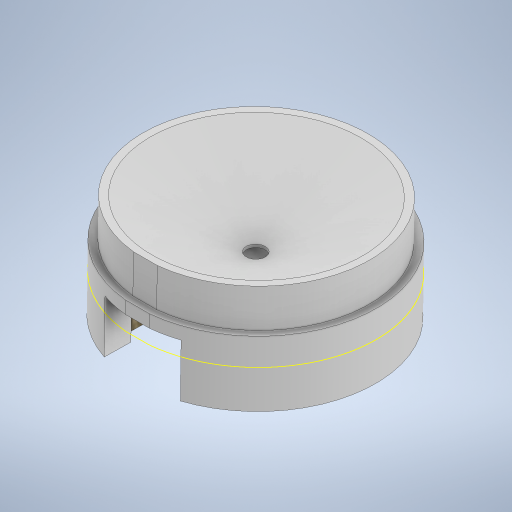
# Autodesk Inventor part: PiezoMount
Saved by Autodesk Inventor 2023 (Build 270158000, 158)
## iProperties
Created: 2023-02-27
Part Number: PiezoMount
Material: Generic
Document SubType Name: Modeling
Designer: maste
Density: 1 g/cm^3
Appearance: Default
Author: maste
Autodesk Inventor part; units mm, degrees
ref_plane "YZ Plane" through (0, 0, 0) normal (1, 0, 0) x (0, 1, 0)
ref_plane "XY Plane" through (0, 0, 0) normal (0, 0, 1) x (1, 0, 0)
sketch "Sketch1" plane through (0, 0, 0) normal (0, 0, 1) x (1, 0, 0)
  circle A0 centre (0, 0) radius 25
  dimension "d2" = 50
  constraints: 1 centre point, 1 coincident
  measures "d2" diameter of A0
extrude "piezo surface" add sketch "Sketch1" along normal blind 8
sketch "Sketch4" plane through (0, 0, 0) normal (0, 0, -1) x (-1, 0, 0)
  circle A0 centre (0, 0) radius 25 projected
extrude "Depth extension to surface" add sketch "Sketch4" along normal blind 3.62
sketch "Sketch2" plane through (0, 0, 8) normal (0, 0, 1) x (1, 0, 0)
  circle A0 centre (0, 0) radius 17.95
  circle A1 centre (0, 0) radius 18.75
  line L0 (0, 0) -> (18.75, 0)
  arc A2 (18.75, 0) -> (16.238, 9.375) centre (0, 0) ccw
  line L1 (0, 0) -> (16.238, 9.375) construction
  line L2 (0, 0) -> (18.75, 0) construction
  line L3 (16.238, 9.375) -> (15.5452, 8.975)
  line L4 (0, 0) -> (0, 18.75)
  line L5 (0, 0) -> (0, -18.75)
  line L6 (0, 0) -> (-18.75, 0)
  line L7 (0, 0) -> (-16.238, -9.375)
  line L8 (0, 0) -> (-9.375, 16.238)
  line L9 (0, 0) -> (9.375, -16.238)
  point P0 (17.95, 0)
  point P1 (8.975, -15.5452)
  point P2 (0, -17.95)
  point P3 (-15.5452, -8.975)
  point P4 (-17.95, 0)
  point P5 (-8.975, 15.5452)
  point P6 (0, 17.95)
  dimension "d3" = 35.9
  dimension "d4" = 37.5
  dimension "d5" = 30
  constraints: 20 end point, 4 point on line, 3 coincident, 2 perpendicular, 2 point on circle, 1 centre point, 1 horizontal, 1 vertical, 12 other
  measures "d5" angle of L2 L1
sketch "Sketch3" plane through (0, 0, 8) normal (0, 0, 1) x (1, 0, 0)
  line L0 (0, 0) -> (8.975, -15.5452)
  arc A0 (17.95, 0) -> (15.5452, 8.975) centre (0, 0) ccw projected
  line L1 (0, 0) -> (17.95, 0)
  arc A1 (0, -17.95) -> (8.975, -15.5452) centre (0, 0) ccw projected
  line L2 (8.975, -15.5452) -> (17.95, 0)
  line L3 (13.4625, -7.7726) -> (0, 0)
  line L4 (13.4625, -7.7726) -> (4.8022, -2.7726)
  line L5 (13.4625, -7.7726) -> (4.8022, -2.7726)
  line L6 (13.4625, -7.7726) -> (4.8022, -2.7726)
  line L7 (4.8022, -2.7726) -> (6.0522, -0.6075)
  line L8 (6.0522, -0.6075) -> (14.7125, -5.6075)
  line L9 (14.7125, -5.6075) -> (13.4625, -7.7726)
  line L10 (13.4625, -7.7726) -> (4.8022, -2.7726)
  line L11 (4.8022, -2.7726) -> (3.5522, -4.9376)
  line L12 (3.5522, -4.9376) -> (12.2125, -9.9376)
  line L13 (12.2125, -9.9376) -> (13.4625, -7.7726)
  line L14 (12.2125, -9.9376) -> (14.7125, -5.6075)
  line L15 (14.7125, -5.6075) -> (16.4446, -6.6075)
  line L16 (16.4446, -6.6075) -> (13.9446, -10.9376)
  line L17 (13.9446, -10.9376) -> (12.2125, -9.9376)
  line L18 (-4.802, 2.7724) -> (-3.552, 4.9375)
  line L19 (-3.552, 4.9375) -> (-13.9443, 10.9375)
  line L20 (-4.802, 2.7724) -> (-6.052, 0.6074)
  line L21 (-6.052, 0.6074) -> (-16.4443, 6.6074)
  line L22 (-16.4443, 6.6074) -> (-23.8055, 10.8574)
  line L23 (-23.8055, 10.8574) -> (-21.3055, 15.1875)
  line L24 (-21.3055, 15.1875) -> (-13.9443, 10.9375)
  line L25 (-5.5448, 2.5) -> (-17.5448, 2.5)
  line L26 (-5.5448, 0) -> (-5.5448, 2.5)
  line L27 (-5.5448, 0) -> (-5.5448, -2.5)
  line L28 (-5.5448, -2.5) -> (-17.5448, -2.5)
  line L29 (-17.5448, -2.5) -> (-26.0448, -2.5)
  line L30 (-26.0448, -2.5) -> (-26.0448, 2.5)
  line L31 (-26.0448, 2.5) -> (-17.5448, 2.5)
  point P0 (14.7125, -5.6075)
  point P1 (12.2125, -9.9376)
  point P2 (12.2125, -9.9376)
  dimension "d37" = 10
  dimension "d38" = 2.5
  dimension "d39" = 2.5
  dimension "d40" = 2
  dimension "d49" = 10
  dimension "d69" = 30
  dimension "d71" = 20.5
  dimension "d72" = 5
  constraints: 64 end point, 7 parallel, 4 collinear, 3 perpendicular, 1 midpoint, 1 point on line, 15 other
  measures "d37" distance of L3.start L4.end
  measures "d38" distance of L4.end L7.end
  measures "d39" distance of L11.end L4.end
  measures "d40" distance of L8.end L15.end
  measures "d49" distance between parallel lines of L11 L13
  measures "d71" distance between parallel lines of L30 L27
  measures "d72" distance between parallel lines of L25 L28
extrude "Microphone Wire Hole" cut sketch "Sketch3" against normal blind 14 contours L26 L27 L28 L29 L30 L31 L25 L21 L20 | L20 L21 L25 L26
sketch "Sketch5" plane through (0, 0, -3.62) normal (0, 0, -1) x (-1, 0, 0)
  line L0 (16, -16) -> (-16, -16)
  line L1 (-16, -16) -> (-16, 16)
  line L2 (-16, 16) -> (16, 16)
  line L3 (16, 16) -> (16, -16)
  line L4 (16, -16) -> (-16, 16) construction
  line L5 (-16, -16) -> (16, 16) construction
  circle A0 centre (0, 0) radius 20
  point P0 (-12, -16)
  point P1 (12, -16)
  point P2 (-16, 12)
  point P3 (-16, -12)
  point P4 (16, 12)
  point P5 (16, -12)
  point P6 (12, 16)
  point P7 (-12, 16)
  dimension "d18" = 32
  dimension "d19" = 32
  dimension "d54" = 40
  constraints: 12 end point, 2 midpoint, 2 parallel, 1 centre point, 1 coincident, 1 horizontal, 1 perpendicular
  measures "d18" distance of L0.start L0.end
  measures "d19" distance of L0.end L1.end
  measures "d54" diameter of A0
extrude "Circuit chamber" cut sketch "Sketch5" against normal blind 3
sketch "Sketch6" plane through (-16, -16, -3.62) normal (1, 0, 0) x (0, 0, -1)
  line L0 (0, 4) -> (0, 0) projected
  line L1 (0, 32) -> (-3, 32) projected
  line L2 (-3, 32) -> (-3, 28) projected
  line L3 (0, 0) -> (-3, 0) projected
  line L4 (-3, 4) -> (-3, 0) projected
  line L5 (0, 32) -> (0, 28) projected
  line L6 (0, 4) -> (-3, 4) projected
  line L7 (0, 18.5) -> (0, 13.5) projected
  line L8 (-11.62, 13.5) -> (-11.62, 18.5) projected
  line L9 (-3, 32) -> (-3, 28) projected
  line L10 (-3, 32) -> (-3, 32) projected
  line L11 (-3, 28) -> (-3, 32) projected
  line L12 (-3, 4) -> (-3, 28) projected
  line L13 (-3, 0) -> (-3, 4) projected
  line L14 (-3, 0) -> (-3, 0) projected
  line L15 (-3, 4) -> (-3, 0) projected
  line L16 (-3, 13.5) -> (-3, 4) projected
  line L17 (0, 18.5) -> (0, 13.5) projected
  line L18 (0, 13.5) -> (0, 4) projected
  line L19 (0, 4) -> (0, 0) projected
  line L20 (0, 0) -> (0, 0) projected
  line L21 (0, 0) -> (0, 4) projected
  line L22 (0, 4) -> (0, 28) projected
  line L23 (0, 28) -> (0, 32) projected
  line L24 (0, 32) -> (0, 32) projected
  line L25 (0, 32) -> (0, 28) projected
  line L26 (-11.62, 16) -> (0, 16)
  line L27 (0, 16) -> (-3, 16)
  line L28 (-3, 16) -> (-3, 24)
  line L29 (-3, 24) -> (0, 24)
  line L30 (0, 24) -> (0, 16)
  line L31 (0, 16) -> (-3, 16)
  line L32 (-3, 16) -> (-3, 8)
  line L33 (-3, 8) -> (0, 8)
  line L34 (0, 8) -> (0, 16)
  line L35 (0, 28) -> (0, 18.5) projected
  line L36 (-3, 18.5) -> (-3, 13.5) projected
  line L37 (-3, 28) -> (-3, 18.5) projected
  line L38 (0, 28) -> (-3, 28) projected
  line L39 (0, 18.5) -> (-11.62, 18.5) projected
  line L40 (-11.62, 13.5) -> (0, 13.5) projected
  point P0 (0, -9)
  point P1 (0, 41)
  point P2 (-11, 41)
  point P3 (-11, -9)
  point P4 (0, -9)
  point P5 (0, 41)
  point P6 (-3, 4)
  point P7 (-3, 8)
  point P8 (0, 8)
  point P9 (-3, 16)
  point P10 (-3, 13.5)
  point P11 (0, 13.5)
  point P12 (0, 18.5)
  dimension "d65" = 8
  dimension "d66" = 8
  constraints: 18 end point, 4 parallel, 2 horizontal, 2 midpoint, 2 perpendicular, 2 point on line
  measures "d65" distance of L27.end L28.end
  measures "d66" distance of L32.end L31.end
extrude "port vent" cut sketch "Sketch6" against normal blind 30 contours L33 L12 L40 L18 | L39 L12 L29 L22
sketch "Sketch7" plane through (0, 0, -3.62) normal (0, 0, -1) x (-1, 0, 0)
  line L0 (0, 0) -> (0, -17.5)
  line L1 (0, 0) -> (0, 17.5)
  dimension "d25" = 17.5
  dimension "d26" = 17.5
  constraints: 4 end point, 2 coincident, 2 vertical
  measures "d25" distance of L0.start L0.end
  measures "d26" distance of L0.start L1.end
hole "screw holes" at (0, 17.5, -3.62) at (0, -17.5, -3.62) direction (0, 0, 1) diameter 3.7 depth 4 tip angle 118
sketch "Sketch8" plane through (0, 0, -3.62) normal (0, 0, -1) x (-1, 0, 0)
  circle A0 centre (0, 0) radius 22.75
  line L0 (21.4137, 11) -> (22.4499, 11) projected
  line L1 (22.4499, 11) -> (19.9139, 11)
  arc A1 (23.6854, 8) -> (23.6854, -8) centre (0, 0) ccw projected
  line L2 (24.6779, -4) -> (22.3956, -4)
  arc A2 (24.8747, 2.5) -> (24.8747, -2.5) centre (0, 0) ccw projected
  arc A3 (-16, 12) -> (-16, -12) centre (0, 0) ccw projected
  arc A4 (-12, -16) -> (12, -16) centre (0, 0) ccw projected
  point P0 (12.5, 7.5)
  point P1 (15.0629, 9)
  point P2 (19.2094, 16)
  point P3 (19.2094, -16)
  point P4 (19.9139, 11)
  point P5 (16.7033, 11)
  point P6 (24.6779, 4)
  point P7 (21.9317, -12)
  dimension "d34" = 45.5
  constraints: 4 end point, 2 point on circle, 1 centre point, 1 coincident, 1 horizontal, 1 parallel, 1 other
  measures "d34" diameter of A0
sketch "Sketch10" plane through (0, 0, -3.62) normal (0, 0, -1) x (-1, 0, 0)
  arc A0 (23.6854, 8) -> (23.6854, -8) centre (0, 0) ccw projected
  arc A1 (16, -12) -> (18.3303, -8) centre (0, 0) ccw projected
  line L0 (16, -16) -> (12, -16) projected
  arc A2 (-12, -16) -> (12, -16) centre (0, 0) ccw projected
  line L1 (-12, -16) -> (-16, -16) projected
  line L2 (-16, -16) -> (-16, -12) projected
  arc A3 (-16, 12) -> (-16, -12) centre (0, 0) ccw projected
  line L3 (-16, 12) -> (-16, 16) projected
  line L4 (-16, 16) -> (-12, 16) projected
  arc A4 (12, 16) -> (-12, 16) centre (0, 0) ccw projected
  line L5 (12, 16) -> (16, 16) projected
  line L6 (16, 16) -> (16, 12) projected
  line L7 (18.3303, 8) -> (23.6854, 8) projected
  line L8 (23.6854, -8) -> (18.3303, -8) projected
  line L9 (16, -12) -> (16, -16) projected
  arc A5 (18.3303, 8) -> (16, 12) centre (0, 0) ccw projected
extrude "Base Extension" add sketch "Sketch10" along normal blind 10
sketch "Sketch13" plane through (0, 0, 8) normal (0, 0, 1) x (0, 1, 0)
  circle A0 centre (0, 0) radius 25
  circle A1 centre (0, 0) radius 23.5
  dimension "d55" = 47
  dimension "d59" = 50
  constraints: 2 centre point, 2 coincident
  measures "d55" diameter of A1
  measures "d59" diameter of A0
extrude "Rim for flush with diaphragm lock" cut sketch "Sketch13" against normal blind 8
sketch "Sketch14" plane through (-16, 12.1244, -3) normal (1, 0, 0) x (0, 0, -1)
  line L0 (10.62, -4.1244) -> (10.62, -20.1244) projected
  line L1 (-3, 11.3756) -> (-11, 11.3756) projected
  line L2 (-11, 11.3756) -> (-11, -35.6244) projected
  line L3 (-3, -9.6244) -> (-3, -14.6244) projected
  line L4 (-2.38, -20.1244) -> (10.62, -20.1244) projected
  line L5 (10.62, -4.1244) -> (-2.38, -4.1244) projected
  line L6 (-3, -14.6244) -> (-2.38, -14.6244) projected
  line L7 (-2.38, -14.6244) -> (-2.38, -20.1244) projected
  line L8 (-2.38, -4.1244) -> (-2.38, -9.6244) projected
  line L9 (-2.38, -9.6244) -> (-3, -9.6244) projected
  point P0 (-3, -12.1244)
  point P1 (-4, -2.6061)
  point P2 (-4, 1.724)
  point P3 (-11, -35.6244)
  constraints: 1 other
sketch "Sketch16" plane through (0, 0, 8) normal (0, 0, 1) x (1, 0, 0)
  circle A0 centre (0, 0) radius 18
  arc A1 (-23.3666, -2.5) -> (-23.3666, 2.5) centre (0, 0) ccw projected
  line L0 (-23.3666, 2.5) -> (-5.5448, 2.5) projected
  line L1 (-5.5448, 2.5) -> (-5.5448, -2.5) projected
  line L2 (-5.5448, -2.5) -> (-23.3666, -2.5) projected
  point P0 (-17.8255, -2.5)
  point P1 (-17.8255, 2.5)
  dimension "d73" = 36
  constraints: 1 centre point, 1 coincident
  measures "d73" diameter of A0
extrude "Extrusion11" add sketch "Sketch16" along normal blind 1 contours A0 L2 L1 L0 picked at (2.3035, 0)
sketch "Sketch17" plane through (0, 0, -13.62) normal (0, 0, -1) x (-1, 0, 0)
  arc A0 (12, 16) -> (-12, 16) centre (0, 0) ccw projected
  line L0 (12, 16) -> (-12, 16)
  line L1 (-12, 20.5) -> (12, 20.5)
  line L2 (12, 20.5) -> (12, 11.5)
  line L3 (12, 11.5) -> (-12, 11.5)
  line L4 (-12, 11.5) -> (-12, 20.5)
  line L5 (-12, 20.5) -> (12, 11.5) construction
  line L6 (12, 20.5) -> (-12, 11.5) construction
  arc A1 (-16, 12) -> (-16, -12) centre (0, 0) ccw projected
  line L7 (0, 0) -> (-20, 0)
  line L8 (-12, -20.5) -> (12, -20.5)
  line L9 (12, -20.5) -> (12, -11.5)
  line L10 (12, -11.5) -> (-12, -11.5)
  line L11 (-12, -11.5) -> (-12, -20.5)
  point P0 (0, 16)
  dimension "d76" = 9
  constraints: 24 end point, 4 symmetric about line, 3 midpoint, 2 parallel, 1 horizontal, 1 perpendicular, 1 point on circle
  measures "d76" distance of L1.end L2.end
extrude "Extrusion12" add sketch "Sketch17" against normal blind 4
fillet "Fillet1" radius 5 4 edges at (-12, -11.5, -11.62) (12, -11.5, -11.62) (12, 11.5, -11.62) (-12, 11.5, -11.62)
sketch "Sketch18" plane through (0, 0, -13.62) normal (0, 0, -1) x (-1, 0, 0)
  circle A0 centre (0, -17.5) radius 1.85 projected
  circle A1 centre (0, 17.5) radius 1.85 projected
  arc A2 (23.6854, 8) -> (23.6854, -8) centre (0, 0) ccw projected
  dimension "d87" = 17.5
  dimension "d88" = 17.5
  dimension "d92" = 3.7
  measures "d87" distance of A2.centre A1.centre
  measures "d88" distance of point (0, 0) A0.centre
  measures "d92" diameter of A0
extrude "Extrusion13" cut sketch "Sketch18" against normal blind 4
sketch "Sketch19" plane through (0, 0, -9.62) normal (0, 0, 1) x (1, 0, 0)
  circle A0 centre (0, 17.5) radius 1.85 projected
  arc A1 (-12, 16) -> (-7.0251, 11.5) centre (-7.0251, 16.5) ccw projected
  line L0 (-7.0251, 11.5) -> (7.0251, 11.5) projected
  arc A2 (7.0251, 11.5) -> (12, 16) centre (7.0251, 16.5) ccw projected
  arc A3 (12, 16) -> (-12, 16) centre (0, 0) ccw projected
  line L1 (-1.2512, 20.6061) -> (2.0643, 20.1366)
  circle A4 centre (0, -17.5) radius 1.85 projected
  arc A5 (12, -16) -> (7.0251, -11.5) centre (7.0251, -16.5) ccw projected
  line L2 (7.0251, -11.5) -> (-7.0251, -11.5) projected
  arc A6 (-7.0251, -11.5) -> (-12, -16) centre (-7.0251, -16.5) ccw projected
  arc A7 (-12, -16) -> (12, -16) centre (0, 0) ccw projected
  circle A8 centre (0, -17.5) radius 1.85 projected
  line L3 (3.5218, -17.5) -> (1.7609, -20.55)
  line L4 (1.7609, -20.55) -> (-1.7609, -20.55)
  line L5 (-1.7609, -20.55) -> (-3.5218, -17.5)
  line L6 (-3.5218, -17.5) -> (-1.7609, -14.45)
  line L7 (-1.7609, -14.45) -> (1.7609, -14.45)
  line L8 (1.7609, -14.45) -> (3.5218, -17.5)
  line L9 (1.7609, 20.55) -> (3.5218, 17.5)
  line L10 (3.5218, 17.5) -> (1.7609, 14.45)
  line L11 (1.7609, 14.45) -> (-1.7609, 14.45)
  line L12 (-1.7609, 14.45) -> (-3.5218, 17.5)
  line L13 (-3.5218, 17.5) -> (-1.7609, 20.55)
  line L14 (-1.7609, 20.55) -> (1.7609, 20.55)
  point P0 (-2.1451, -19.8846)
  point P1 (2.1451, -19.8846)
  dimension "d83" = 6.1
  dimension "d86" = 6.1
  dimension "d209" = 0
  constraints: 26 end point, 3 coincident, 28 other
  measures "d83" distance between parallel lines of L6 L3
  measures "d86" distance between parallel lines of L12 L9
  measures "d209" angle of L2 L7
extrude "Extrusion14" cut sketch "Sketch19" against normal blind 1 contours A0 | L13 L14 L1 L9 A3 | A3 L9 L10 L11 L12 L13 | L1 L14 L9 | L3 L4 L5 A7 | A7 L5 L6 L7 L8 L3
sketch "Sketch20" plane through (0, 0, -0.62) normal (0, 0, -1) x (-1, 0, 0)
  circle A0 centre (0, 17.5) radius 1.85 projected
  line L0 (-1.7609, 14.45) -> (1.7609, 14.45) projected
  line L1 (-3.5218, 17.5) -> (-1.7609, 14.45) projected
  line L2 (-1.7609, 20.55) -> (-3.5218, 17.5) projected
  line L3 (1.7609, 20.55) -> (-1.7609, 20.55) projected
  line L4 (3.5218, 17.5) -> (1.7609, 20.55) projected
  line L5 (1.7609, 14.45) -> (3.5218, 17.5) projected
  line L6 (1.7609, -14.45) -> (-1.7609, -14.45) projected
  line L7 (3.5218, -17.5) -> (1.7609, -14.45) projected
  line L8 (1.7609, -20.55) -> (3.5218, -17.5) projected
  line L9 (-3.5218, -17.5) -> (-1.7609, -20.55) projected
  line L10 (-1.7609, -14.45) -> (-3.5218, -17.5) projected
  circle A1 centre (0, -17.5) radius 1.85 projected
  line L11 (-1.7609, -20.55) -> (1.7609, -20.55) projected
  point P0 (0, 0)
  dimension "d91" = 6.1
  measures "d91" distance between parallel lines of L9 L7
extrude "Extrusion15" cut sketch "Sketch20" along normal blind 11 contours L1 L2 L3 L4 L5 L0 | L7 L8 L11 L9 L10 L6 | A1
ref_plane "Work Plane3" through (0, 23.5, 0) normal (0, 1, 0) x (-1, 0, 0)
sketch "Sketch28" plane through (0, 0, -13.62) normal (0, 0, -1) x (-1, 0, 0)
  point P0 (0, 0)
sketch "Sketch27" plane through (0, 0, -0.62) normal (0, 0, -1) x (-1, 0, 0)
  circle A0 centre (0, 17.5) radius 1.85 projected
  circle A1 centre (0, -17.5) radius 1.85 projected
  arc A2 (7.0251, 11.5) -> (12, 16) centre (7.0251, 16.5) ccw projected
  line L0 (12, 16) -> (16, 16) projected
  line L1 (16, 16) -> (16, 12) projected
  arc A3 (18.3303, 8) -> (16, 12) centre (0, 0) ccw projected
  line L2 (18.3303, 8) -> (23.6854, 8) projected
  arc A4 (23.6854, 8) -> (23.6854, -8) centre (0, 0) ccw projected
  line L3 (23.6854, -8) -> (18.3303, -8) projected
  arc A5 (16, -12) -> (18.3303, -8) centre (0, 0) ccw projected
  line L4 (16, -12) -> (16, -16) projected
  line L5 (16, -16) -> (12, -16) projected
  arc A6 (12, -16) -> (7.0251, -11.5) centre (7.0251, -16.5) ccw projected
  line L6 (7.0251, -11.5) -> (-7.0251, -11.5) projected
  arc A7 (-7.0251, -11.5) -> (-12, -16) centre (-7.0251, -16.5) ccw projected
  line L7 (-12, -16) -> (-16, -16) projected
  line L8 (-16, -16) -> (-16, -12) projected
  arc A8 (-16, 12) -> (-16, -12) centre (0, 0) ccw projected
  line L9 (-16, 12) -> (-16, 16) projected
  line L10 (-16, 16) -> (-12, 16) projected
  arc A9 (-12, 16) -> (-7.0251, 11.5) centre (-7.0251, 16.5) ccw projected
  line L11 (-7.0251, 11.5) -> (7.0251, 11.5) projected
  line L12 (18.3303, 8) -> (-3.4197, 8)
  line L13 (-3.4197, 8) -> (-3.4197, -8)
  line L14 (-3.4197, -8) -> (18.3303, -8)
  line L15 (18.3303, -8) -> (18.3303, 8)
  line L16 (-3.4197, 0) -> (16.0803, 0)
  line L17 (16.0803, 0) -> (16.0803, 10)
  line L18 (16.0803, 10) -> (-3.4197, 10)
  line L19 (-3.4197, 10) -> (-3.4197, 0)
  line L20 (-3.4197, 0) -> (16.0803, 0)
  line L21 (16.0803, 0) -> (16.0803, -10)
  line L22 (16.0803, -10) -> (-3.4197, -10)
  line L23 (-3.4197, -10) -> (-3.4197, 0)
  line L24 (20.3303, -11.5) -> (20.3303, 11.5)
  line L25 (20.3303, 11.5) -> (-7.6697, 11.5)
  line L26 (-7.6697, 11.5) -> (-7.6697, -11.5)
  line L27 (-7.6697, -11.5) -> (20.3303, -11.5)
  line L28 (20.3303, -11.5) -> (-7.6697, 11.5) construction
  line L29 (20.3303, 11.5) -> (-7.6697, -11.5) construction
  point P0 (6.3303, 0)
  point P1 (-7.0251, -11.5)
  point P2 (16.3631, -11.5)
  point P3 (17.3205, -10)
  point P4 (17.3205, 10)
  point P5 (16.3631, 11.5)
  point P6 (16.0803, 8)
  point P7 (16.0803, -8)
  point P8 (20.3303, 8)
  point P9 (20.3303, -8)
  dimension "d132" = 21.75
  dimension "d133" = 16
  dimension "d134" = 10
  dimension "d135" = 10
  dimension "d136" = 28
  constraints: 36 end point, 8 parallel, 4 midpoint, 4 perpendicular, 3 horizontal, 1 point on line, 1 vertical
  measures "d132" distance of L14.end L13.end
  measures "d133" distance of L14.end L2.start
  measures "d134" distance of L17.end L16.end
  measures "d135" distance of L20.end L21.end
  measures "d136" distance of L25.end L24.end
extrude "Extrusion20" add sketch "Sketch27" along normal blind 5 contours L25 A3 L12 L17 L18 L19 L13 L23 L22 L21 L14 A5 L27 L6 L26 L11 | A2 L0 L1 A3 L25 | L25 L24 L2 A3 | L3 L24 L27 A5
sketch "Sketch30" plane through (0, 0, -0.62) normal (0, 0, -1) x (-1, 0, 0)
  line L0 (16.0803, 10) -> (-3.4197, 10) projected
  line L1 (-3.4197, 10) -> (-3.4197, -10) projected
  line L2 (-3.4197, -10) -> (16.0803, -10) projected
  arc A0 (12, 16) -> (2.1451, 19.8846) centre (0, 0) ccw projected
  line L3 (16.0803, -8) -> (23.6854, -8) projected
  line L4 (5.5448, -2.5) -> (24.8747, -2.5) projected
  line L5 (5.5448, 2.5) -> (5.5448, -2.5) projected
  line L6 (24.8747, 2.5) -> (5.5448, 2.5) projected
  line L7 (23.6854, 8) -> (16.0803, 8) projected
  arc A1 (-12, -16) -> (-2.1451, -19.8846) centre (0, 0) ccw projected
  arc A2 (23.6854, -8) -> (24.8747, -2.5) centre (0, 0) ccw projected
  arc A3 (24.8747, 2.5) -> (23.6854, 8) centre (0, 0) ccw projected
  line L8 (16.3631, -11.5) -> (-7.6697, -11.5) projected
  line L9 (-7.6697, -11.5) -> (-7.6697, 11.5) projected
  line L10 (-7.6697, 11.5) -> (7.0251, 11.5) projected
  arc A4 (7.0251, 11.5) -> (12, 16) centre (7.0251, 16.5) ccw projected
  line L11 (2.1451, 19.8846) -> (1.7609, 20.55) projected
  line L12 (1.7609, 20.55) -> (-1.7609, 20.55) projected
  line L13 (-1.7609, 20.55) -> (-2.1451, 19.8846) projected
  arc A5 (2.1451, -19.8846) -> (12, -16) centre (0, 0) ccw projected
  line L14 (-16, 16) -> (-12, 16) projected
  line L15 (-16, 12) -> (-16, 16) projected
  line L16 (-16, -16) -> (-16, -12) projected
  line L17 (-12, -16) -> (-16, -16) projected
  arc A6 (-2.1451, 19.8846) -> (-12, 16) centre (0, 0) ccw projected
  line L18 (-2.1451, -19.8846) -> (-1.7609, -20.55) projected
  line L19 (-1.7609, -20.55) -> (1.7609, -20.55) projected
  line L20 (1.7609, -20.55) -> (2.1451, -19.8846) projected
  arc A7 (-16, 12) -> (-16, -12) centre (0, 0) ccw projected
  line L21 (16, -16) -> (12, -16) projected
  line L22 (16, -12) -> (16, -16) projected
  arc A8 (16, -12) -> (16.3631, -11.5) centre (0, 0) ccw projected
  line L23 (16.0803, 8) -> (16.0803, 10) projected
  line L24 (16.0803, -10) -> (16.0803, -8) projected
extrude "Extrusion21" add sketch "Sketch30" along normal blind 2 contours L23 L7 A3 L6 L5 L4 A2 L3 L24 L2 L1 L0
sketch "Sketch31" plane through (0, 0, 9) normal (0, 0, 1) x (1, 0, 0)
  circle A0 centre (0, 0) radius 2
  dimension "d153" = 4
  constraints: 1 centre point, 1 coincident
  measures "d153" diameter of A0
extrude "Extrusion22" cut sketch "Sketch31" against normal blind 15
chamfer "Chamfer10" distance 0.5 angle 45 2 edges at (0, 14.45, -9.62) (0, -14.45, -9.62)
chamfer "Chamfer11" distance 0.5 angle 45 8 edges at (-1.6166, -14.2, -9.62) (-2.6414, -15.975, -9.62) (1.6166, -14.2, -9.62) (2.6414, -15.975, -9.62) (-1.6166, 14.2, -9.62) (-2.6414, 15.975, -9.62) (1.6166, 14.2, -9.62) (2.6414, 15.975, -9.62)
sketch "Sketch49" plane through (0, 0, -5.62) normal (0, 0, -1) x (-1, 0, 0)
  line L0 (17.5701, -10.7544) -> (5.518, -10.7544)
  line L1 (5.518, -10.7544) -> (5.518, -16.7393)
  line L2 (5.518, -16.7393) -> (17.5701, -16.7393)
  line L3 (17.5701, -16.7393) -> (17.5701, -10.7544)
  point P0 (0, 0)
  constraints: 8 end point, 2 parallel, 1 horizontal, 1 perpendicular
extrude "Extrusion37" add sketch "Sketch49" against normal blind 2.97
sketch "Sketch50" plane through (0, 0, -9.62) normal (0, 0, 1) x (1, 0, 0)
  arc A0 (12, 16) -> (2.1451, 19.8846) centre (0, 0) ccw projected
  line L0 (2.1451, 19.8846) -> (4.6765, 15.5) projected
  line L1 (4.6765, 15.5) -> (3.7816, 13.95) projected
  line L2 (7.0251, 11.5) -> (-2.0496, 11.5) projected
  arc A1 (7.0251, 11.5) -> (12, 16) centre (7.0251, 16.5) ccw projected
  line L3 (-2.0496, -11.5) -> (7.0251, -11.5) projected
  line L4 (3.7816, -13.95) -> (4.6765, -15.5) projected
  line L5 (4.6765, -15.5) -> (2.1451, -19.8846) projected
  arc A2 (2.1451, -19.8846) -> (12, -16) centre (0, 0) ccw projected
  arc A3 (12, -16) -> (7.0251, -11.5) centre (7.0251, -16.5) ccw projected
  line L6 (7.6697, -11.5) -> (-5.518, -11.5) projected
  line L7 (7.6697, -2.275) -> (7.6697, -11.5) projected
  arc A4 (3.4197, -7.2323) -> (7.6697, -2.275) centre (0, 0) ccw projected
  line L8 (3.4197, -10) -> (3.4197, -7.2323) projected
  line L9 (-16.0803, -10) -> (3.4197, -10) projected
  line L10 (-16.0803, -8) -> (-16.0803, -10) projected
  line L11 (-23.6854, -8) -> (-16.0803, -8) projected
  arc A5 (-23.6854, -8) -> (-23.6854, 8) centre (0, 0) ccw projected
  line L12 (-16.0803, 8) -> (-23.6854, 8) projected
  line L13 (-16.0803, 10) -> (-16.0803, 8) projected
  line L14 (3.4197, 10) -> (-16.0803, 10) projected
  line L15 (3.4197, 7.2323) -> (3.4197, 10) projected
  arc A6 (7.6697, 2.275) -> (3.4197, 7.2323) centre (0, 0) ccw projected
  line L16 (7.6697, 11.5) -> (7.6697, 2.275) projected
  line L17 (-7.0251, 11.5) -> (7.6697, 11.5) projected
  arc A7 (-12, 16) -> (-7.0251, 11.5) centre (-7.0251, 16.5) ccw projected
  arc A8 (-2.1451, 19.8846) -> (-12, 16) centre (0, 0) ccw projected
  line L18 (-1.7609, 20.55) -> (-2.1451, 19.8846) projected
  line L19 (1.7609, 20.55) -> (-1.7609, 20.55) projected
  line L20 (2.1451, 19.8846) -> (1.7609, 20.55) projected
  arc A9 (12, 16) -> (2.1451, 19.8846) centre (0, 0) ccw projected
  line L21 (16, 16) -> (12, 16) projected
  line L22 (16, 12) -> (16, 16) projected
  arc A10 (16, -12) -> (16, 12) centre (0, 0) ccw projected
  line L23 (16, -16) -> (16, -12) projected
  line L24 (12, -16) -> (16, -16) projected
  arc A11 (2.1451, -19.8846) -> (12, -16) centre (0, 0) ccw projected
  line L25 (1.7609, -20.55) -> (2.1451, -19.8846) projected
  line L26 (-1.7609, -20.55) -> (1.7609, -20.55) projected
  line L27 (-2.1451, -19.8846) -> (-1.7609, -20.55) projected
  arc A12 (-10.9452, -16.7393) -> (-2.1451, -19.8846) centre (0, 0) ccw projected
  line L28 (-10.9452, -16.7393) -> (-5.518, -16.7393) projected
  line L29 (-5.518, -16.7393) -> (-5.518, -11.5) projected
  line L30 (7.0251, 11.5) -> (-2.0496, 11.5) projected
  line L31 (-2.0496, 13.95) -> (-2.0496, 11.5) projected
  arc A13 (2.1451, -19.8846) -> (12, -16) centre (0, 0) ccw projected
  arc A14 (2.1451, -19.8846) -> (12, -16) centre (0, 0) ccw projected
  line L32 (-2.0496, -11.5) -> (-2.0496, -13.95) projected
  line L33 (-2.0496, -11.5) -> (7.0251, -11.5) projected
  line L34 (-4.6765, 15.5) -> (4.8497, 15.5)
  line L35 (4.8497, 15.5) -> (4.8497, 10)
  line L36 (4.8497, 10) -> (-4.6765, 10)
  line L37 (-4.6765, 10) -> (-4.6765, 15.5)
  line L38 (-16.0803, -10) -> (3.4197, -10) projected
  line L39 (4.6765, -15.5) -> (-4.6765, -15.5)
  line L40 (-4.6765, -15.5) -> (-4.6765, -10)
  line L41 (-4.6765, -10) -> (4.6765, -10)
  line L42 (4.6765, -10) -> (4.6765, -15.5)
  line L43 (-2.0496, -11.5) -> (7.0251, -11.5) projected
  line L44 (-2.0496, -11.5) -> (-2.0496, -13.95) projected
  line L45 (-2.0496, -13.95) -> (3.7816, -13.95) projected
  line L46 (3.7816, -13.95) -> (4.6765, -15.5) projected
  line L47 (4.6765, -15.5) -> (2.1451, -19.8846) projected
  arc A15 (12, -16) -> (7.0251, -11.5) centre (7.0251, -16.5) ccw projected
  arc A16 (12, 16) -> (2.1451, 19.8846) centre (0, 0) ccw projected
  line L48 (2.1451, 19.8846) -> (4.6765, 15.5) projected
  line L49 (4.6765, 15.5) -> (3.7816, 13.95) projected
  line L50 (3.7816, 13.95) -> (-2.0496, 13.95) projected
  arc A17 (7.0251, 11.5) -> (12, 16) centre (7.0251, 16.5) ccw projected
  line L51 (-2.0496, -11.5) -> (-2.0496, -13.95) projected
  line L52 (-2.0496, -13.95) -> (3.7816, -13.95) projected
  line L53 (3.7816, 13.95) -> (-2.0496, 13.95) projected
  line L54 (-2.0496, 13.95) -> (-2.0496, 11.5) projected
  line L55 (-2.0496, -13.95) -> (3.7816, -13.95) projected
  line L56 (3.7816, -13.95) -> (4.6765, -15.5) projected
  line L57 (4.6765, -15.5) -> (2.1451, -19.8846) projected
  arc A18 (12, -16) -> (7.0251, -11.5) centre (7.0251, -16.5) ccw projected
  arc A19 (12, 16) -> (2.1451, 19.8846) centre (0, 0) ccw projected
  line L58 (2.1451, 19.8846) -> (4.6765, 15.5) projected
  line L59 (4.6765, 15.5) -> (3.7816, 13.95) projected
  line L60 (3.7816, 13.95) -> (-2.0496, 13.95) projected
  line L61 (-2.0496, 13.95) -> (-2.0496, 11.5) projected
  line L62 (7.0251, 11.5) -> (-2.0496, 11.5) projected
  arc A20 (7.0251, 11.5) -> (12, 16) centre (7.0251, 16.5) ccw projected
  point P0 (-2.0496, -11.5)
  point P1 (-4.6765, -11.5)
  point P2 (4.6765, -11.5)
  point P3 (-4.6765, 11.5)
  point P4 (-2.0496, 11.5)
  point P5 (4.8497, 11.5)
  point P6 (4.6765, -11.5)
  point P7 (12, -16)
  point P8 (2.1451, 19.8846)
  point P9 (4.8497, 11.5)
  point P10 (-4.6765, 10)
  point P11 (2.1451, 19.8846)
  constraints: 16 end point, 4 parallel, 2 horizontal, 2 perpendicular, 2 point on line
extrude "Extrusion38" cut sketch "Sketch50" along normal blind 7 contours A1 L2 L35 L34 L0 A0 | L0 L34 L37 L17 A7 A8 L18 L19 L20 | L34 L35 L2 L31 L50 L1 | L1 L50 L31 L17 L37 L34 | L35 L36 L14 L37 L17 L2 | A2 L5 L42 L3 A3 | L25 L26 L27 A12 L28 L29 L6 L40 L39 L5 | L39 L40 L6 L32 L45 L4 | L4 L45 L32 L3 L42 | L3 L6 L40 L9 L41 L42
sketch "Sketch51" plane through (0, 0, -5.62) normal (0, 0, -1) x (-1, 0, 0)
  line L0 (-3.4197, -10) -> (-3.4197, 10) projected
  line L1 (4.6765, 10) -> (16.0803, 10) projected
  line L2 (16.0803, 10) -> (16.0803, 8) projected
  line L3 (16.0803, 8) -> (18.3303, 8) projected
  arc A0 (18.3303, 8) -> (16, 12) centre (0, 0) ccw projected
  line L4 (16, 16) -> (16, 12) projected
  line L5 (12, 16) -> (16, 16) projected
  arc A1 (7.0251, 11.5) -> (12, 16) centre (7.0251, 16.5) ccw projected
  line L6 (7.0251, 11.5) -> (4.6765, 11.5) projected
  line L7 (-7.6697, 11.5) -> (-7.6697, -11.5) projected
  line L8 (-7.6697, -11.5) -> (-4.6765, -11.5) projected
  line L9 (16, -16) -> (12, -16) projected
  line L10 (16, -12) -> (16, -16) projected
  arc A2 (16, -12) -> (18.3303, -8) centre (0, 0) ccw projected
  line L11 (18.3303, -8) -> (16.0803, -8) projected
  line L12 (16.0803, -8) -> (16.0803, -10) projected
  line L13 (16.0803, -10) -> (4.6765, -10) projected
  line L14 (-3.4197, -10) -> (-3.4197, 10) projected
  line L15 (-7.6697, 11.5) -> (-7.6697, -11.5) projected
  line L16 (4.6765, 11.5) -> (4.6765, 15.5) projected
  line L17 (4.6765, 15.5) -> (4.6765, 11.5) projected
  line L18 (-4.8497, 15.5) -> (-4.8497, 11.5) projected
  line L19 (-4.8497, 11.5) -> (-4.8497, 15.5) projected
  line L20 (-4.6765, -11.5) -> (-4.6765, -15.5) projected
  line L21 (-4.6765, -15.5) -> (-4.6765, -11.5) projected
  line L22 (4.6765, -15.5) -> (4.6765, -11.5) projected
  line L23 (4.6765, -11.5) -> (4.6765, -15.5) projected
  line L24 (-7.6697, 2.275) -> (-7.6697, 10)
  line L25 (-4.6765, -15.5) -> (-4.8497, 11.5)
  line L26 (-4.8497, 11.5) -> (-4.8497, 11.5)
  line L27 (4.6765, -11.5) -> (4.6765, -10)
  line L28 (4.6765, 11.5) -> (4.6765, 10)
  line L29 (4.6765, 10) -> (16.0803, 10) projected
  line L30 (16.0803, 10) -> (16.0803, 8) projected
  line L31 (16.0803, 8) -> (18.3303, 8) projected
  arc A3 (18.3303, 8) -> (16, 12) centre (0, 0) ccw projected
  line L32 (16, 16) -> (16, 12) projected
  line L33 (12, 16) -> (16, 16) projected
  arc A4 (7.0251, 11.5) -> (12, 16) centre (7.0251, 16.5) ccw projected
  line L34 (7.0251, 11.5) -> (4.6765, 11.5) projected
  line L35 (-7.6697, -11.5) -> (-4.6765, -11.5) projected
  line L36 (16, -16) -> (12, -16) projected
  line L37 (16, -12) -> (16, -16) projected
  arc A5 (16, -12) -> (18.3303, -8) centre (0, 0) ccw projected
  line L38 (18.3303, -8) -> (16.0803, -8) projected
  line L39 (16.0803, -8) -> (16.0803, -10) projected
  line L40 (16.0803, -10) -> (4.6765, -10) projected
  line L41 (5.518, -11.5) -> (5.518, -16.7393) projected
  line L42 (5.518, -16.7393) -> (10.9452, -16.7393) projected
  arc A6 (10.9452, -16.7393) -> (12, -16) centre (0, 0) ccw projected
  line L43 (5.518, -11.5) -> (5.518, -16.7393) projected
  line L44 (5.518, -16.7393) -> (10.9452, -16.7393) projected
  arc A7 (10.9452, -16.7393) -> (12, -16) centre (0, 0) ccw projected
  line L45 (4.6765, 11.5) -> (4.6765, 10) projected
  line L46 (4.6765, -10) -> (4.6765, -11.5) projected
  line L47 (4.6765, -11.5) -> (5.518, -11.5) projected
  line L48 (-3.4197, 10) -> (-4.8497, 10) projected
  line L49 (-4.8497, 10) -> (-4.8497, 11.5) projected
  line L50 (-4.8497, 11.5) -> (-7.6697, 11.5) projected
  line L51 (-4.6765, -11.5) -> (-4.6765, -10) projected
  line L52 (-4.6765, -10) -> (-3.4197, -10) projected
  line L53 (4.6765, 11.5) -> (4.6765, 10) projected
  line L54 (4.6765, -10) -> (4.6765, -11.5) projected
  line L55 (4.6765, -11.5) -> (5.518, -11.5) projected
  line L56 (-3.4197, 10) -> (-4.8497, 10) projected
  line L57 (-4.8497, 10) -> (-4.8497, 11.5) projected
  line L58 (-4.8497, 11.5) -> (-7.6697, 11.5) projected
  line L59 (-4.6765, -11.5) -> (-4.6765, -10) projected
  line L60 (-4.6765, -10) -> (-3.4197, -10) projected
  point P0 (-4.7022, -11.5)
  point P1 (-4.8497, 11.5)
  point P2 (-4.7022, -11.5)
  point P3 (-4.8497, 11.5)
  point P4 (-4.8497, 11.5)
  point P5 (-4.8401, 10)
  point P6 (-4.8497, 11.5)
  point P7 (-4.8497, 11.5)
  point P8 (-4.8401, 10)
  constraints: 10 end point, 4 point on line, 2 perpendicular
extrude "Extrusion39" add sketch "Sketch51" along normal blind 8
chamfer "Chamfer12" distance 2 angle 45 2 edges at (-16.0803, -8, -8.12) (-16.0803, 8, -8.12)
sketch "Sketch52" plane through (0, 0, -2.62) normal (0, 0, -1) x (-1, 0, 0)
  line L0 (18.0803, 8) -> (16.0803, 10) projected
  line L1 (18.0803, 8) -> (14.0803, 8)
  line L2 (14.0803, 8) -> (14.0803, -8)
  line L3 (14.0803, -8) -> (18.0803, -8)
  line L4 (18.0803, -8) -> (18.0803, 8)
  point P0 (0, 0)
  dimension "d230" = 4
  constraints: 8 end point, 2 parallel, 1 horizontal, 1 perpendicular
  measures "d230" distance of L3.end L2.end
extrude "Extrusion40" add sketch "Sketch52" along normal blind 2.5
sketch "Sketch53" plane through (0, 0, 9) normal (0, 0, 1) x (1, 0, 0)
  circle A0 centre (0, 0) radius 2 projected
  line L0 (-5.5448, -2.5) -> (-17.8255, -2.5) projected
  arc A1 (-17.8255, -2.5) -> (-17.8255, 2.5) centre (0, 0) ccw projected
  line L1 (-17.8255, 2.5) -> (-5.5448, 2.5) projected
  line L2 (-5.5448, 2.5) -> (-5.5448, -2.5) projected
extrude "Extrusion41" cut sketch "Sketch53" against normal blind 1
sketch "Sketch54" plane through (0, 0, -13.62) normal (0, 0, -1) x (-1, 0, 0)
  line L0 (-3.4197, -10) -> (-3.4197, 10) projected
  line L1 (-3.4197, -10) -> (4.5803, -10)
  line L2 (4.5803, -10) -> (4.5803, 10)
  line L3 (4.5803, 10) -> (-3.4197, 10)
  line L4 (-3.4197, 10) -> (-3.4197, -10)
  line L5 (4.5803, -10) -> (-3.4197, -10)
  line L6 (-3.4197, -10) -> (-3.4197, -12)
  line L7 (-3.4197, -12) -> (4.5803, -12)
  line L8 (4.5803, -12) -> (4.5803, -10)
  line L9 (4.5803, 10) -> (-3.4197, 10)
  line L10 (-3.4197, 10) -> (-3.4197, 12)
  line L11 (-3.4197, 12) -> (4.5803, 12)
  line L12 (4.5803, 12) -> (4.5803, 10)
  point P0 (0, 0)
  point P1 (-3.4197, 10)
  dimension "d233" = 8
  dimension "d234" = 2
  dimension "d235" = 2
  constraints: 24 end point, 6 parallel, 3 horizontal, 3 perpendicular, 2 point on line
  measures "d233" distance of L3.end L2.end
  measures "d234" distance of L6.end L5.end
  measures "d235" distance of L9.end L10.end
extrude "Extrusion42" cut sketch "Sketch54" against normal blind 10 contours L1 L8 L7 L6 | L10 L11 L12 L3
sketch "Sketch55" plane through (-23.3666, 2.5, 8) normal (0, -1, 0) x (1, 0, 0)
  line L0 (0, 0) -> (17.8218, 0) projected
  line L1 (0, 0) -> (0, -8) projected
  line L2 (0, -8) -> (-1.508, -8) projected
  line L3 (-1.508, -10.62) -> (-1.508, -8) projected
  line L4 (5.2863, -10.62) -> (-1.508, -10.62) projected
  line L5 (9.2863, -10.62) -> (5.2863, -10.62) projected
  line L6 (17.8218, -10.62) -> (9.2863, -10.62) projected
  line L7 (17.8218, 0) -> (17.8218, -10.62) projected
  point P0 (23.3666, -8)
extrude "Extrusion43" add sketch "Sketch55" along normal blind 5
chamfer "Chamfer13" distance 10 distance2 20 1 edges at (-2, 0, 8) measured on face at (-2, 0, 7.5)
sketch "Sketch56" plane through (0, 0, -0.62) normal (0, 0, -1) x (-1, 0, 0)
  circle A0 centre (0, -17.5) radius 1.85 projected
  circle A1 centre (0, 17.5) radius 1.85 projected
  line L0 (16.3631, -11.5) -> (-7.6697, -11.5) projected
  line L1 (-7.6697, -11.5) -> (-7.6697, 11.5) projected
  line L2 (-7.6697, 11.5) -> (7.0251, 11.5) projected
  arc A2 (7.0251, 11.5) -> (12, 16) centre (7.0251, 16.5) ccw projected
  arc A3 (12, 16) -> (2.1451, 19.8846) centre (0, 0) ccw projected
  line L3 (2.1451, 19.8846) -> (1.7609, 20.55) projected
  line L4 (1.7609, 20.55) -> (-1.7609, 20.55) projected
  line L5 (-1.7609, 20.55) -> (-2.1451, 19.8846) projected
  arc A4 (-2.1451, 19.8846) -> (-12, 16) centre (0, 0) ccw projected
  line L6 (-16, 16) -> (-12, 16) projected
  line L7 (-16, 12) -> (-16, 16) projected
  arc A5 (-16, 12) -> (-16, -12) centre (0, 0) ccw projected
  line L8 (-16, -16) -> (-16, -12) projected
  line L9 (-12, -16) -> (-16, -16) projected
  arc A6 (-12, -16) -> (-2.1451, -19.8846) centre (0, 0) ccw projected
  line L10 (-2.1451, -19.8846) -> (-1.7609, -20.55) projected
  line L11 (-1.7609, -20.55) -> (1.7609, -20.55) projected
  line L12 (1.7609, -20.55) -> (2.1451, -19.8846) projected
  arc A7 (2.1451, -19.8846) -> (12, -16) centre (0, 0) ccw projected
  line L13 (16, -16) -> (12, -16) projected
  line L14 (16, -12) -> (16, -16) projected
  arc A8 (16, -12) -> (16.3631, -11.5) centre (0, 0) ccw projected
  line L15 (4.5803, 11.5) -> (4.5803, 12) projected
  line L16 (4.5803, 11.5) -> (-3.4197, 11.5)
  line L17 (-3.4197, 11.5) -> (-3.4197, 22.5)
  line L18 (-3.4197, 22.5) -> (4.5803, 22.5)
  line L19 (4.5803, 22.5) -> (4.5803, 11.5)
  line L20 (4.5803, -11.5) -> (-3.4197, -11.5)
  line L21 (-3.4197, -11.5) -> (-3.4197, -22.5)
  line L22 (-3.4197, -22.5) -> (4.5803, -22.5)
  line L23 (4.5803, -22.5) -> (4.5803, -11.5)
  dimension "d243" = 8
  dimension "d244" = 11
  dimension "d245" = 11
  constraints: 16 end point, 4 parallel, 3 point on line, 2 horizontal, 2 perpendicular
  measures "d243" distance of L17.end L18.end
  measures "d244" distance of L16.end L17.end
  measures "d245" distance of L21.end L20.end
extrude "Extrusion44" add sketch "Sketch56" along normal blind 5 contours A0 | A1 | L23 A7 L12 L11 L10 A6 L21 L0 | L23 L22 L21 A6 L10 L11 L12 A7 | L17 A4 L5 L4 L3 A3 L19 L15 L2 | L17 L18 L19 A3 L3 L4 L5 A4
sketch "Sketch58" plane through (0, 0, -5.62) normal (0, 0, -1) x (-1, 0, 0)
  arc A0 (23.6854, 8) -> (23.6854, -8) centre (0, 0) ccw projected
  line L0 (24.8747, 2.5) -> (24.8747, -2.5) projected
  arc A1 (24.8747, 2.5) -> (24.8747, -2.5) centre (0, 0) ccw projected
sketch "Sketch59" plane through (0, 0, -9.62) normal (0, 0, 1) x (1, 0, 0)
  line L0 (4.8497, 11.5) -> (10.4112, 11.5)
  line L1 (10.4112, 11.5) -> (10.4112, 21.3262)
  line L2 (10.4112, 21.3262) -> (4.8497, 21.3262)
  line L3 (4.8497, 21.3262) -> (4.8497, 11.5)
  line L4 (4.7022, -11.5) -> (9.6436, -11.5)
  line L5 (9.6436, -11.5) -> (9.6436, -20.5106)
  line L6 (9.6436, -20.5106) -> (4.7022, -20.5106)
  line L7 (4.7022, -20.5106) -> (4.7022, -11.5)
  line L8 (-5.518, -16.7393) -> (-11.6107, -16.7393)
  line L9 (-11.6107, -16.7393) -> (-11.6107, -20.5106)
  line L10 (-11.6107, -20.5106) -> (-5.518, -20.5106)
  line L11 (-5.518, -20.5106) -> (-5.518, -16.7393)
  line L12 (-7.0251, 11.5) -> (-4.6765, 11.5) projected
  line L13 (-4.6765, 11.5) -> (-12.6182, 11.5)
  line L14 (-12.6182, 11.5) -> (-12.6182, 20.0308)
  line L15 (-12.6182, 20.0308) -> (-4.6765, 20.0308)
  line L16 (-4.6765, 20.0308) -> (-4.6765, 11.5)
  point P0 (0, 0)
  constraints: 32 end point, 8 parallel, 4 horizontal, 4 perpendicular, 1 point on line
extrude "Extrusion46" add sketch "Sketch59" along normal blind 4
body "Solid1"
